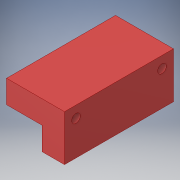
# Autodesk Inventor part: КВ33.044.502 - Фиксатор оси Y
Saved by Autodesk Inventor 2019 (Build 230136000, 136)
## iProperties
Created: 2019-08-02
Part Number: КВ33.044.502 - Фиксатор оси Y
Material: Пластик АБС
Document SubType Name: Modeling
Designer: Петров Иван
Density: 1.06 g/cm^3
Appearance: Гладкий — красный
Author: Петров Иван
Autodesk Inventor part; units mm, degrees
ref_plane "YZ Plane" through (0, 0, 0) normal (1, 0, 0) x (0, 1, 0)
ref_plane "XZ Plane" through (0, 0, 0) normal (0, 1, 0) x (-1, 0, 0)
ref_plane "XY Plane" through (0, 0, 0) normal (0, 0, 1) x (1, 0, 0)
sketch "Эскиз1" plane through (0, 0, 0) normal (1, 0, 0) x (0, 1, 0)
  line L0 (-4, 19) -> (4, 19)
  line L1 (4, 19) -> (4, -19)
  line L2 (4, -19) -> (-4, -19)
  line L3 (-4, -19) -> (-4, 19)
  line L4 (-4, 19) -> (4, -19) construction
  line L5 (4, 19) -> (-4, -19) construction
  point P0 (0, 0)
  dimension "d0" = 8
  dimension "d1" = 38
  constraints: 12 end point, 2 midpoint, 2 parallel, 1 horizontal, 1 perpendicular
  measures "d0" distance of L1.end L2.end
  measures "d1" distance of L0.end L1.end
extrude "Выдавливание1" add sketch "Эскиз1" along normal blind 20.2
sketch "Эскиз2" plane through (0, 0, 0) normal (-1, 0, 0) x (0, 0, 1)
  line L0 (0, 0) -> (-15, 0)
  line L1 (0, 0) -> (15, 0) construction
  line L2 (-15, 0) -> (15, 0)
  circle A0 centre (-15, 0) radius 1.5
  circle A1 centre (15, 0) radius 1.5
  dimension "d4" = 15
  dimension "d5" = 180
  dimension "d6" = 30
  dimension "d7" = 3
  dimension "d8" = 3
  constraints: 6 end point, 2 centre point, 2 coincident, 2 horizontal, 1 collinear, 1 point on line
  measures "d4" distance of L0.start L0.end
  measures "d5" angle of L0 L1
  measures "d6" distance of L0.end L2.end
  measures "d7" diameter of A0
  measures "d8" diameter of A1
extrude "Выдавливание2" cut sketch "Эскиз2" against normal through all
sketch "Эскиз3" plane through (0, -4, -19) normal (0, -1, 0) x (1, 0, 0)
  line L0 (0, 38) -> (20.2, 38) projected
  line L1 (0, 0) -> (20.2, 0) projected
  line L2 (20.2, 38) -> (12.4, 38)
  line L3 (12.4, 38) -> (12.4, 0)
  line L4 (12.4, 0) -> (20.2, 0)
  line L5 (20.2, 0) -> (20.2, 38)
  point P0 (0, 19)
  dimension "d11" = 7.8
  constraints: 8 end point, 2 parallel, 1 horizontal, 1 perpendicular, 1 point on line
  measures "d11" distance of L4.end L3.end
extrude "Выдавливание3" add sketch "Эскиз3" along normal blind 8
